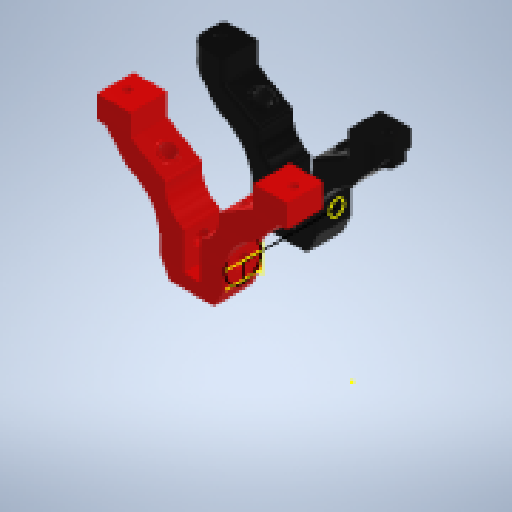
# Autodesk Inventor part: LR2_X_mount
Saved by Autodesk Inventor 2023 (Build 270158000, 158)
## iProperties
Created: 2023-11-24
Part Number: LR2_X_mount
Material: Generic
Document SubType Name: Modeling
Designer: danie
Density: 1 g/cm^3
Appearance: Default
Author: danie
Autodesk Inventor part; units mm, degrees
ref_plane "YZ Plane" through (0, 0, 0) normal (1, 0, 0) x (0, 1, 0)
ref_plane "XZ Plane" through (0, 0, 0) normal (0, 1, 0) x (-1, 0, 0)
ref_plane "Work Plane1" through (0, 0, 50) normal (0, 0, 1) x (1, 0, 0)
sketch "Sketch1" plane through (0, 0, 50) normal (0, 0, 1) x (1, 0, 0)
  line L0 (78.5048, 100.9746) -> (78.5048, 75.6677) projected
  line L1 (74.1646, 106.6483) -> (78.5048, 100.9746) projected
  line L2 (66.7714, 110.9168) -> (74.1646, 106.6483) projected
  line L3 (66.7714, 118.1168) -> (66.7714, 110.9168) projected
  line L4 (69.2037, 122.3297) -> (66.7714, 118.1168) projected
  arc A0 (71.9358, 123.0617) -> (69.2037, 122.3297) centre (70.9358, 121.3297) ccw projected
  line L5 (86.9326, 114.4033) -> (71.9358, 123.0617) projected
  arc A1 (87.9173, 112.4242) -> (86.9326, 114.4033) centre (85.9326, 112.6712) ccw projected
  arc A2 (87.9173, 112.4242) -> (96.4441, 97.2164) centre (102.5048, 110.6089) ccw projected
  arc A3 (98.0048, 94.7971) -> (96.4441, 97.2164) centre (95.3493, 94.7971) ccw projected
  line L6 (98.0048, 75.6677) -> (98.0048, 94.7971) projected
  line L7 (98.0048, 75.6677) -> (78.5048, 75.6677) projected
  line L8 (120.1048, 75.6677) -> (120.1048, 87.6659) projected
  line L9 (120.1048, 75.6677) -> (107.0048, 75.6677) projected
  line L10 (107.0048, 94.7727) -> (107.0048, 75.6677) projected
  arc A4 (108.5843, 97.2249) -> (107.0048, 94.7727) centre (109.6982, 94.7727) ccw projected
  arc A5 (108.5843, 97.2249) -> (117.0923, 112.4242) centre (102.5048, 110.6089) ccw projected
  arc A6 (118.077, 114.4033) -> (117.0923, 112.4242) centre (119.077, 112.6712) ccw projected
  line L11 (133.0738, 123.0617) -> (118.077, 114.4033) projected
  arc A7 (135.8059, 122.3297) -> (133.0738, 123.0617) centre (134.0738, 121.3297) ccw projected
  line L12 (138.2382, 118.1168) -> (135.8059, 122.3297) projected
  line L13 (138.2382, 110.9168) -> (138.2382, 118.1168) projected
  line L14 (131.1521, 106.8256) -> (138.2382, 110.9168) projected
  arc A8 (131.1521, 106.8256) -> (120.1048, 87.6659) centre (146.6818, 85.1066) ccw projected
  line L15 (107.0048, 75.6677) -> (98.0048, 75.6677)
  line L16 (119.9126, 78.6076) -> (115.5557, 69.2642)
  arc A9 (113.7431, 68.1094) -> (115.5557, 69.2642) centre (113.7431, 70.1094) ccw
  line L17 (115.5557, 69.2642) -> (113.7431, 70.1094) construction
  line L18 (113.7431, 68.1094) -> (113.7431, 70.1094) construction
  line L19 (113.7431, 68.1094) -> (102.5048, 68.1094)
  line L20 (102.5048, 68.1094) -> (102.5048, 75.6677)
  arc A10 (119.9126, 78.6076) -> (120.1, 79.4528) centre (118.1001, 79.4528) ccw
  line L21 (120.1, 79.4528) -> (120.1048, 87.6659)
  line L22 (138.2382, 110.9168) -> (138.3644, 110.9931)
  arc A11 (138.3644, 110.9931) -> (138.8916, 111.4336) centre (137.1967, 112.9258) ccw
  line L23 (138.8916, 111.4336) -> (149.722, 124.2405)
  line L24 (149.722, 124.2405) -> (154.4624, 124.2405)
  line L25 (133.0738, 123.0617) -> (136.122, 124.8216)
  line L26 (149.722, 124.2405) -> (149.722, 136.8926)
  line L27 (149.722, 136.8926) -> (136.122, 136.8926)
  line L28 (136.122, 136.8926) -> (136.122, 124.8216)
  line L29 (149.722, 136.8926) -> (154.4624, 136.8926)
  line L30 (154.4624, 136.8926) -> (154.4624, 124.2405)
  line L31 (154.4624, 124.2405) -> (149.722, 124.2405)
  line L32 (149.722, 124.2405) -> (149.722, 136.8926)
  point P0 (0, 0)
  point P1 (120.1, 88.8376)
  point P2 (118.5417, 75.6677)
  dimension "d8" = 2
  dimension "d10" = 13.6
  constraints: 36 end point, 6 point on circle, 5 tangent, 3 centre point, 3 horizontal, 3 perpendicular, 2 parallel, 1 collinear, 1 midpoint, 1 vertical
  measures "d8" radius of A9
  measures "d10" distance of L26.end L27.end
extrude "Extrusion1" add sketch "Sketch1" along normal blind 20 contours L21 A10 L16 L9 L10 A4 A5 A6 L11 A7 L12 L13 L14 A8 | L16 A9 L19 L20 L15 L9 | L13 L12 A7 L25 L28 L27 L26 L23 A11 L22 | L26 L29 L30 L24
sketch "Sketch3" plane through (149.722, 124.2405, 50) normal (0, -1, 0) x (1, 0, 0)
  circle A0 centre (-1.7192, -41.2716) radius 1.9956 projected
  line L0 (0, 0) -> (0, 20) projected
  line L1 (0, 10) -> (-38, 10)
  line L2 (-1.7192, -41.2716) -> (-1.7192, 10)
  circle A1 centre (-1.7192, 10) radius 6
  line L3 (0, 20) -> (-5.8867, 14.3165)
  line L4 (0, 0) -> (-5.8867, 5.6835)
  point P0 (-149.722, -50)
  point P1 (0, 15.7484)
  point P2 (0, 4.2516)
  dimension "d13" = 12
  constraints: 8 end point, 2 coincident, 2 point on circle, 2 tangent, 1 centre point, 1 horizontal, 1 midpoint, 1 perpendicular, 1 point on line
  measures "d13" diameter of A1
extrude "Extrusion2" cut sketch "Sketch3" along normal blind 20 contours L4 L2 A1 L0 | A1 L2 L1 L0 | L0 A1 | L4 A1 L2 | L1 A1 L0 | A1 L1 L2 | A1 L3 L0
hole "Hole1" at (148.0028, 124.2405, 60) direction (0, 1, 0) diameter 4 end through all clearance for "Countersunk Flat Head Screw ISO 2009/7046" size "M4" standard "ISO"
sketch "Sketch4" plane through (138.2382, 110.9168, 50) normal (0.4999997, -0.8660256, 0) x (0.8660256, 0.4999997, 0)
  line L0 (20.7125, 0) -> (20.7125, 20) projected
  line L1 (20.7125, 10) -> (-35.121, 10)
  line L2 (-35.121, 0) -> (-35.121, 20) projected
  ellipse E0 centre (-7.6054, -41.2727) end of major axis (-4.2155, -38.9714) minor radius 4.0972 projected
  line L3 (-7.6054, -41.2727) -> (-7.2042, 10)
  circle A0 centre (-7.2042, 10) radius 10
  line L4 (-8.1823, 20) -> (0, 20) projected
  point P0 (-175.1762, -50)
  constraints: 4 end point, 3 midpoint, 2 coincident, 1 centre point, 1 tangent
extrude "Extrusion3" cut sketch "Sketch4" along normal blind 20 contours A0 L3 L1 | L1 A0 | L3 A0 L1
hole "Hole2" at (131.9991, 107.3147, 60) direction (-0.4999997, 0.8660256, 0) diameter 8 end through all clearance for "Slotted Cheese Head Screw ISO 1207" size "M8" standard "ISO"
sketch "Sketch5" plane through (120.1048, 87.6659, 70) normal (0.9999998, -0.0005825, 0) x (0, 0, -1)
  ellipse E0 centre (61.2749, -0.5565) end of major axis (57.175, -0.5565) minor radius 4.0999 projected
  line L0 (20, 0) -> (0, 0) projected
  line L1 (10, 0) -> (10, -9.0584)
  line L2 (20, -9.0584) -> (0, -9.0584) projected
  line L3 (61.2749, -0.5565) -> (10, -0.5565)
  circle A0 centre (10, -0.5565) radius 10
  line L4 (20, 7.0991) -> (20, -12.0059) projected
  point P0 (70, -87.7358)
  constraints: 4 end point, 2 midpoint, 1 centre point, 1 coincident, 1 perpendicular, 1 point on line, 1 tangent, 1 other
extrude "Extrusion4" cut sketch "Sketch5" along normal blind 20 contours A0 L3 L1 L0 | L0 A0 | A0 L2 L1 L3 | L1 L2 A0 L0 | A0 L2
sketch "Sketch6" plane through (118.077, 114.4033, 70) normal (-0.5000004, 0.8660252, 0) x (0.8660252, 0.5000004, 0)
  circle A0 centre (8.5127, 10) radius 4 projected
  line L0 (20.8366, 20) -> (0, 20) projected
  line L1 (0, 20) -> (0, 0) projected
  line L2 (20.8366, 0) -> (0, 0) projected
  line L3 (20.8366, 20) -> (20.8366, 0) projected
  circle A1 centre (8.5127, 10) radius 6
  point P0 (-159.4593, 70)
  dimension "d41" = 2
  constraints: 1 centre point
  measures "d41" radial gap between concentric circles of A0 A1
extrude "Extrusion5" add sketch "Sketch6" along normal blind 1 contours A1
sketch "Sketch7" plane through (107.0048, 75.6677, 50) normal (-1, 0.0000001, 0) x (0, 0, 1)
  line L0 (0, 19.105) -> (0, 0) projected
  line L1 (0, 0) -> (20, 0) projected
  line L2 (20, 19.105) -> (20, 0) projected
  line L3 (0, 19.105) -> (20, 19.105) projected
  ellipse E0 centre (10, 11.4493) end of major axis (10, 17.4493) minor radius 6
  point P0 (-50, -75.6677)
  constraints: 2 other
fillet "Fillet1" radius 1 1 edges at (119.753, 116.5256, 60) inverted yes
mirror "Mirror2" about plane through (102.5048, 75.6677, 50) normal (-1, 0, 0)
extrude "Extrusion7" add sketch "Sketch7" along normal blind 1 contours E0
fillet "Fillet2" radius 1 1 edges at (106.0048, 81.117, 60) inverted yes
hole "Hole5" at (120.1045, 87.1094, 60) direction (-0.9999998, 0.0005825, 0) diameter 8 depth 35.1993 tip angle 118 clearance for "Countersunk Flat Head Screw ISO 2009/7046" size "M8" standard "ISO"
body "Solid1"
